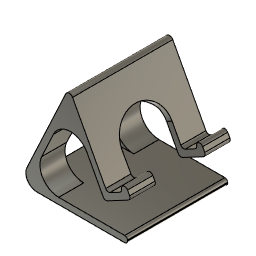
PhoneStand v1 (Autodesk Fusion 360 design; units mm, degrees)
Autodesk Fusion 360 part; units mm, degrees
note: some values were not read from the file. Set by a fixed rule: which sketch regions a step uses.
sketch "Schizzo1" plane through (0, 0, 0) normal (0, 0, 1) x (1, 0, 0)
  line L0 (0, 0) -> (90, 0)
  line L1 (90, 0) -> (90, 80)
  line L2 (90, 80) -> (0, 80)
  line L3 (0, 80) -> (0, 0)
  dimension "d1" = 90
  dimension "d2" = 80
  constraint horizontal L0
  constraint vertical L1
  constraint horizontal L2
  constraint vertical L3
  constraint coincident L0.start L3.end
  measures "d1" distance of L1.end L2.end
  measures "d2" distance of L0.start L2.end
extrude "Estrusione1" add sketch "Schizzo1" along normal blind 85
sketch "Schizzo2" plane through (0, 0, 0) normal (0, -1, 0) x (1, 0, 0)
  line L0 (0, 0) -> (90, 0)
  line L1 (90, 0) -> (90, 85)
  line L2 (90, 85) -> (0, 85)
  line L3 (0, 85) -> (0, 0)
  line L4 (90, 0) -> (90, 5)
  line L5 (90, 5) -> (0, 5)
  line L6 (0, 5) -> (0, 0)
  line L7 (0, 0) -> (90, 0)
  line L8 (0, 5) -> (37.3046, 85)
  line L9 (0, 5) -> (76.1109, 5) construction
  line L10 (37.3046, 85) -> (67.8203, 27.6084)
  line L11 (67.8203, 27.6084) -> (80.1815, 34.181)
  line L12 (80.1815, 34.181) -> (77.8342, 38.5957)
  line L13 (4.5315, 2.8869) -> (37.5979, 73.798)
  line L14 (37.5979, 73.798) -> (65.7529, 20.8463)
  line L15 (65.7529, 20.8463) -> (86.9436, 32.1136)
  line L16 (86.9436, 32.1136) -> (82.2489, 40.9431)
  line L17 (77.8342, 38.5957) -> (82.2489, 40.9431)
  line L18 (0, 5) -> (-2.3315, 0)
  line L19 (0, 0) -> (-2.3315, 0)
  dimension "d5" = 5
  dimension "d6" = 65
  dimension "d8" = 53
  dimension "d9" = 65
  dimension "d10" = 14
  dimension "d11" = 5
  dimension "d12" = 5
  constraint coincident L0.end L1.start
  constraint perpendicular L0 L4
  constraint coincident L3 L5.end
  constraint perpendicular L3 L5
  constraint coincident L0.start L3.end
  constraint horizontal L9
  constraint coincident L2 L8.end
  constraint perpendicular L10 L11
  constraint perpendicular L11 L12
  constraint parallel L8 L18
  constraint perpendicular L3 L19
  measures "d5" distance of L0.end L4.end
  measures "d6" angle of L8 L9
  measures "d8" angle of L8 L10
  measures "d9" distance of L8.end L10.end
  measures "d10" distance of L10.end L11.end
  measures "d11" distance of L11.end L12.end
extrude "Estrusione2" cut sketch "Schizzo2" against normal blind 80 contours L2 L3 L8 | L1 L2 L5 L10 L11 L12 L13 L14 L15 L16 L17
fillet "Raccordo1" radius 15 1 edges at (5.5169, 40, 5)
fillet "Raccordo2" radius 15 1 edges at (37.5979, 40, 73.798)
fillet "Raccordo3" radius 2.6 6 edges at (80.1815, 40, 34.181) (77.8342, 40, 38.5957) (82.2489, 40, 40.9431) (67.8203, 40, 27.6084) (86.9436, 40, 32.1136) (65.7529, 40, 20.8463)
fillet "Raccordo4" radius 3 1 edges at (37.3046, 40, 85)
sketch "Schizzo3" plane through (0, 0, 0) normal (0, -1, 0) x (1, 0, 0)
  arc A0 (15.4676, 26.3393) -> (29.0622, 5) centre (29.0622, 20) ccw
  line L0 (15.4676, 26.3393) -> (24.8833, 46.5315)
  arc A1 (51.7222, 47.2343) -> (24.8833, 46.5315) centre (38.4779, 40.1922) ccw
  line L1 (51.7222, 47.2343) -> (64.5323, 23.142)
  arc A2 (64.5323, 23.142) -> (68.0485, 22.0669) centre (66.8279, 24.3626) ccw
  line L2 (68.0485, 22.0669) -> (84.648, 30.893)
  arc A3 (84.648, 30.893) -> (85.723, 34.4093) centre (83.4273, 33.1887) ccw
  line L3 (85.723, 34.4093) -> (84.0462, 37.5629)
  arc A4 (84.0462, 37.5629) -> (79.2079, 35.7992) centre (81.7505, 36.3423) ccw
  arc A5 (77.8859, 32.9604) -> (79.2079, 35.7992) centre (76.6652, 35.256) ccw
  line L4 (77.8859, 32.9604) -> (70.1159, 28.829)
  arc A6 (66.5996, 29.9041) -> (70.1159, 28.829) centre (68.8953, 31.1247) ccw
  line L5 (66.5996, 29.9041) -> (40.1295, 79.6872)
  arc A7 (40.1295, 79.6872) -> (34.7617, 79.5467) centre (37.4806, 78.2788) ccw
  line L6 (34.7617, 79.5467) -> (0, 5)
  line L7 (0, 5) -> (0, 0)
  line L8 (0, 0) -> (90, 0)
  line L9 (0, 5) -> (-2.8175, -1.0421)
  line L10 (0, 0) -> (-2.3315, 0)
  line L11 (90, 0) -> (90, 5)
  line L12 (90, 5) -> (29.0622, 5)
  constraint coincident L6.end L7.start
  constraint parallel L6 L9
  constraint coincident L7.end L8.start
  constraint coincident L9 L10.end
  constraint perpendicular L7 L10
extrude "Estrusione3" add sketch "Schizzo3" against normal blind 80 contours L7 L9 L10
fillet "Raccordo6" radius 9 1 edges at (-2.3315, 40, 0)
sketch "Schizzo4" plane through (0, 0, 0) normal (0, -1, 0) x (1, 0, 0)
  arc A0 (3.6389, 12.8036) -> (11.7956, 0) centre (11.7956, 9) ccw
  line L0 (11.7956, 0) -> (90, 0)
  line L1 (90, 0) -> (90, 5)
  line L2 (90, 5) -> (29.0622, 5)
  arc A1 (15.4676, 26.3393) -> (29.0622, 5) centre (29.0622, 20) ccw
  line L3 (15.4676, 26.3393) -> (24.8833, 46.5315)
  arc A2 (51.7222, 47.2343) -> (24.8833, 46.5315) centre (38.4779, 40.1922) ccw
  line L4 (51.7222, 47.2343) -> (64.5323, 23.142)
  arc A3 (64.5323, 23.142) -> (68.0485, 22.0669) centre (66.8279, 24.3626) ccw
  line L5 (68.0485, 22.0669) -> (84.648, 30.893)
  arc A4 (84.648, 30.893) -> (85.723, 34.4093) centre (83.4273, 33.1887) ccw
  line L6 (85.723, 34.4093) -> (84.0462, 37.5629)
  arc A5 (84.0462, 37.5629) -> (79.2079, 35.7992) centre (81.7505, 36.3423) ccw
  arc A6 (77.8859, 32.9604) -> (79.2079, 35.7992) centre (76.6652, 35.256) ccw
  line L7 (77.8859, 32.9604) -> (70.1159, 28.829)
  arc A7 (66.5996, 29.9041) -> (70.1159, 28.829) centre (68.8953, 31.1247) ccw
  line L8 (66.5996, 29.9041) -> (40.1295, 79.6872)
  arc A8 (40.1295, 79.6872) -> (34.7617, 79.5467) centre (37.4806, 78.2788) ccw
  line L9 (34.7617, 79.5467) -> (3.6389, 12.8036)
  line L10 (100, -5) -> (83.9719, -5)
  line L11 (83.9719, -5) -> (83.9719, 13.2417)
  line L12 (83.9719, 13.2417) -> (100, 13.2417)
  line L13 (100, 13.2417) -> (100, -5)
  constraint horizontal L10
  constraint vertical L11
  constraint horizontal L12
  constraint vertical L13
extrude "Estrusione4" cut sketch "Schizzo4" against normal blind 80 contours L0 L1 L2 L11
fillet "Raccordo7" radius 2.2 2 edges at (83.9719, 40, 5) (83.9719, 40, 0)
sketch "Schizzo5" plane through (64.3166, 0, 34.1978) normal (0.882948, 0, 0.469472) x (0, 1, 0)
  line L0 (80, 51.52) -> (0, 51.52)
  line L1 (0, 51.52) -> (0, -4.8629)
  line L2 (0, -4.8629) -> (80, -4.8629)
  line L3 (80, -4.8629) -> (80, 51.52)
  circle A0 centre (40, 10) radius 20
  line L4 (20.0011, 9.7863) -> (20.3194, -19.9984)
  line L5 (60, 9.9667) -> (59.9501, -19.9992)
  line L6 (59.9501, -19.9992) -> (20.3194, -19.9984)
  line L7 (0, 0) -> (0, 10)
  line L8 (0, 10) -> (40, 10)
  dimension "d34" = 40
  dimension "d39" = 10
  dimension "d40" = 40
  constraint coincident A0 L4.start
  constraint tangent A0 L4
  constraint coincident A0 L5.start
  constraint tangent A0 L5
  constraint coincident L7.start origin
  constraint coincident L1 L7.end
  constraint perpendicular L7 L8
  constraint coincident A0.centre L8.end
  measures "d34" diameter of A0
  measures "d39" distance of L7.start L7.end
  measures "d40" distance of L7.end A0.centre
extrude "Estrusione5" cut sketch "Schizzo5" along normal blind 19 and the other way blind 15 contours L2 A0 L4 L5 L6 | L2 A0 L5 | L2 A0 | L2 A0 | L2 A0 L4
sketch "Schizzo6" plane through (0, 0, 0) normal (1, 0, 0) x (0, 1, 0)
  line L0 (80, 0) -> (80, 5)
  line L1 (80, 5) -> (40, 5)
  line L2 (40, 5) -> (40, 30)
  circle A0 centre (40, 30) radius 20
  line L3 (60, 30) -> (60, 5)
  line L4 (20, 30) -> (20, 5)
  line L5 (20, 5) -> (40, 5)
  dimension "d41" = 5
  dimension "d42" = 40
  dimension "d43" = 25
  dimension "d44" = 40
  constraint vertical L0
  constraint perpendicular L0 L1
  constraint perpendicular L1 L2
  constraint coincident L2.end A0.centre
  constraint coincident A0 L3.start
  constraint midpoint L1 L3.end
  constraint tangent A0 L3
  constraint coincident A0 L4.start
  constraint tangent A0 L4
  constraint vertical L4
  constraint perpendicular L2 L5
  measures "d41" distance of L0.start L0.end
  measures "d42" distance of L0.end L1.end
  measures "d43" distance of L1.end L2.end
  measures "d44" diameter of A0
extrude "Estrusione6" cut sketch "Schizzo6" along normal blind 30
